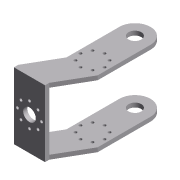
# Autodesk Inventor part: Neck
Saved by Autodesk Inventor 2011 (Build 150239000, 239)
## iProperties
Created: 2010-11-28
Part Number: Neck
Document SubType Name: Modeling
Designer: Milton
Density: 2.71 g/cm^3
Mass: 19.7062 g
Surface Area: 64.3216 cm^2
Volume: 7.27165 cm^3
Material: Aluminum-6061
Author: Milton
Autodesk Inventor part; units mm, degrees
ref_plane "YZ Plane" through (0, 0, 0) normal (1, 0, 0) x (0, 1, 0)
ref_plane "XZ Plane" through (0, 0, 0) normal (0, 1, 0) x (-1, 0, 0)
ref_plane "XY Plane" through (0, 0, 0) normal (0, 0, 1) x (1, 0, 0)
sketch "Sketch1" plane through (0, 0, 0) normal (0, 0, 1) x (1, 0, 0)
  line L0 (9.893, 6.4872) -> (9.893, 9.4872)
  line L1 (31.893, 6.4872) -> (31.893, 9.4872)
  arc A0 (44.393, 68.4872) -> (22.393, 68.4872) centre (33.393, 68.4872) ccw
  line L2 (9.893, 6.4872) -> (31.893, 6.4872)
  line L3 (9.893, 9.4872) -> (22.393, 31.1378)
  line L4 (9.893, 9.4872) -> (39.4953, 9.4872) construction
  line L5 (31.893, 9.4872) -> (44.393, 31.1378)
  line L6 (44.393, 68.4872) -> (44.393, 31.1378)
  line L7 (22.393, 68.4872) -> (22.393, 31.1378)
  circle A1 centre (33.393, 68.4872) radius 4.5
  point P0 (0, 0)
  dimension "d0" = 62
  dimension "d1" = 1.5
  dimension "d2" = 3
  dimension "d3" = 3
  dimension "d5" = 22
  dimension "d6" = 60
  dimension "d7" = 22
  dimension "d8" = 9
  constraints: 16 end point, 2 centre point, 2 horizontal, 2 parallel, 2 perpendicular, 2 point on circle, 2 tangent, 1 coincident, 1 vertical
  measures "d0" distance from line of L2 A0.centre
  measures "d1" distance from line of L1 A0.centre
  measures "d2" distance of L0.start L0.end
  measures "d3" distance of L1.start L1.end
  measures "d5" diameter of A0
  measures "d6" angle of L4 L3
  measures "d7" distance of L0.start L1.start
  measures "d8" diameter of A1
extrude "Extrusion1" add sketch "Sketch1" along normal blind 47
sketch "Sketch2" plane through (9.893, 6.4872, 0) normal (-1, 0, 0) x (0, 0, 1)
  line L0 (0, 3) -> (47, 3) projected
  line L1 (0, 73) -> (47, 73) projected
  line L2 (3, 3) -> (3, 73)
  line L3 (3, 73) -> (44, 73)
  line L4 (44, 73) -> (44, 3)
  line L5 (0, 3) -> (0, 24.6506) projected
  line L6 (47, 24.6506) -> (47, 62) projected
  line L7 (3, 3) -> (44, 3)
  point P0 (0, -6.4872)
  dimension "d11" = 3
  dimension "d12" = 3
  constraints: 8 end point, 3 point on line, 1 parallel
  measures "d11" distance between parallel lines of L5 L2
  measures "d12" distance between parallel lines of L6 L4
extrude "Extrusion2" cut sketch "Sketch2" against normal through all
sketch "Sketch3" plane through (9.893, 6.4872, 0) normal (0, -1, 0) x (1, 0, 0)
  circle A0 centre (11, 23.5) radius 4.5
  line L0 (22, 0) -> (0, 0) projected
  point P0 (-9.893, 0)
  dimension "d15" = 9
  dimension "d18" = 23.5
  constraints: 1 centre point
  measures "d15" diameter of A0
  measures "d18" distance from line of L0 A0.centre
extrude "Extrusion3" cut sketch "Sketch3" against normal through all
sketch "Sketch4" plane through (0, 0, 47) normal (0, 0, 1) x (1, 0, 0)
  circle A0 centre (33.393, 38.4872) radius 4.5
  circle A1 centre (33.393, 46.9872) radius 1
  circle A2 centre (27.3825, 44.4976) radius 1
  circle A3 centre (24.893, 38.4872) radius 1
  circle A4 centre (27.3825, 32.4768) radius 1
  circle A5 centre (33.393, 29.9872) radius 1
  circle A6 centre (39.4034, 32.4768) radius 1
  circle A7 centre (41.893, 38.4872) radius 1
  circle A8 centre (39.4034, 44.4976) radius 1
  point P0 (0, 0)
  constraints: 9 centre point
extrude "Extrusion4" cut sketch "Sketch4" against normal through all contours A1 | A2 | A3 | A4 | A5 | A6 | A7 | A8
sketch "Sketch5" plane through (9.893, 9.4872, 44) normal (0, 1, 0) x (1, 0, 0)
  circle A0 centre (11, 20.5) radius 4.5
  circle A1 centre (11, 29) radius 1
  circle A2 centre (4.9896, 26.5104) radius 1
  circle A3 centre (2.5, 20.5) radius 1
  circle A4 centre (4.9896, 14.4896) radius 1
  circle A5 centre (11, 12) radius 1
  circle A6 centre (17.0104, 14.4896) radius 1
  circle A7 centre (19.5, 20.5) radius 1
  circle A8 centre (17.0104, 26.5104) radius 1
  point P0 (-9.893, 44)
  constraints: 9 centre point
extrude "Extrusion5" cut sketch "Sketch5" against normal through all contours A1 | A2 | A3 | A4 | A5 | A6 | A7 | A8
body "Solid1"
